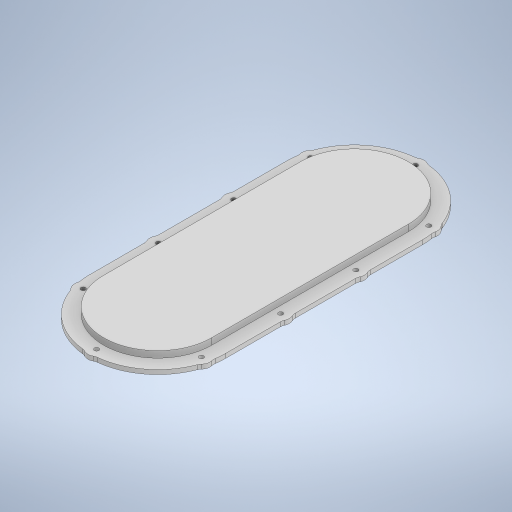
# Autodesk Inventor part: top_housing_bottom_plate
Saved by Autodesk Inventor 2023.1 (Build 271208000, 208)
## iProperties
Created: 2026-04-22
Part Number: top_housing_bottom_plate
Material: Generic
Document SubType Name: Modeling
Designer: Lars
Density: 1 g/cm^3
Appearance: Default
Author: Lars
Autodesk Inventor part; units mm, degrees
ref_plane "YZ Plane" through (0, 0, 0) normal (1, 0, 0) x (0, 1, 0)
ref_plane "XZ Plane" through (0, 0, 0) normal (0, 1, 0) x (-1, 0, 0)
ref_plane "XY Plane" through (0, 0, 0) normal (0, 0, 1) x (1, 0, 0)
sketch "Sketch2" plane through (0, 0, 0) normal (0, 1, 0) x (-1, 0, 0)
  line L0 (15, -6.5) -> (-46, -6.5) construction
  line L1 (-46, -6.5) -> (-46, -90.5) construction
  line L2 (-46, -90.5) -> (15, -90.5) construction
  line L3 (15, -90.5) -> (15, -6.5) construction
  line L4 (46, 27.1) -> (14, 27.1) construction
  line L5 (14, 27.1) -> (14, 11.1) construction
  line L6 (14, 11.1) -> (46, 11.1) construction
  line L7 (46, 11.1) -> (46, 27.1) construction
  line L8 (9, 32.5) -> (-40, 32.5) construction
  line L9 (-40, 32.5) -> (-40, 90.5) construction
  line L10 (-40, 90.5) -> (9, 90.5) construction
  line L11 (9, 90.5) -> (9, 32.5) construction
  line L12 (-15.5, -6.5) -> (-15.5, -90.5) construction
  line L13 (-15.5, 32.5) -> (-15.5, 90.5) construction
  line L14 (-46, -90.5) -> (46, -90.5) construction
  line L15 (46, -90.5) -> (46, 90.5) construction
  line L16 (46, 90.5) -> (-46, 90.5) construction
  line L17 (-46, 90.5) -> (-46, -90.5) construction
  line L18 (46, 0) -> (-46, 0) construction
  line L19 (-62.5, 267) -> (62.5, 267) construction
  line L20 (62.5, 267) -> (62.5, -267) construction
  line L21 (62.5, -267) -> (-62.5, -267) construction
  line L22 (-62.5, -267) -> (-62.5, 267) construction
  line L23 (62.5, 0) -> (-62.5, 0) construction
  circle A0 centre (46, 11.1) radius 1.5
  circle A1 centre (14, 27.1) radius 1.5
  circle A2 centre (9, 32.5) radius 1.5
  circle A3 centre (-40, 32.5) radius 1.5
  circle A4 centre (9, 90.5) radius 1.5
  circle A5 centre (-40, 90.5) radius 1.5
  circle A6 centre (15, -6.5) radius 1.5
  circle A7 centre (15, -90.5) radius 1.5
  circle A8 centre (-46, -90.5) radius 1.5
  circle A9 centre (-46, -6.5) radius 1.5
  line L24 (0, 142) -> (0, 142)
  line L25 (-50, 92) -> (-50, 0)
  line L26 (-50, 0) -> (50, 0) construction
  line L27 (50, 0) -> (50, 92)
  line L28 (50, 0) -> (-50, 0) construction
  line L29 (-50, 0) -> (-50, -90)
  line L30 (0, -140) -> (0, -140)
  line L31 (50, -90) -> (50, 0)
  arc A10 (50, 92) -> (0, 142) centre (0, 92) ccw
  arc A11 (0, 142) -> (-50, 92) centre (0, 92) ccw
  arc A12 (-50, -90) -> (0, -140) centre (0, -90) ccw
  arc A13 (0, -140) -> (50, -90) centre (0, -90) ccw
  line L32 (63, 92) -> (63, 0)
  line L33 (63, 0) -> (63, -90)
  arc A14 (0, -153) -> (63, -90) centre (0, -90) ccw
  arc A15 (-63, -90) -> (0, -153) centre (0, -90) ccw
  line L34 (-63, -90) -> (-63, 0)
  line L35 (-63, 0) -> (-63, 92)
  arc A16 (0, 155) -> (-63, 92) centre (0, 92) ccw
  arc A17 (63, 92) -> (0, 155) centre (0, 92) ccw
  line L36 (56.5, 92) -> (56.5, 0) construction
  line L37 (56.5, 0) -> (56.5, -90) construction
  arc A18 (0, -146.5) -> (56.5, -90) centre (0, -90) ccw construction
  arc A19 (-56.5, -90) -> (0, -146.5) centre (0, -90) ccw construction
  line L38 (-56.5, -90) -> (-56.5, 0) construction
  line L39 (-56.5, 0) -> (-56.5, 92) construction
  arc A20 (0, 148.5) -> (-56.5, 92) centre (0, 92) ccw construction
  arc A21 (56.5, 92) -> (0, 148.5) centre (0, 92) ccw construction
  circle A22 centre (0, -146.5) radius 2.05
  circle A23 centre (0, -146.5) radius 8.05
  circle A24 centre (54.6727, -104.253) radius 2.05
  circle A25 centre (54.6727, -104.253) radius 8.05
  circle A26 centre (56.5, -34.95) radius 2.05
  circle A27 centre (56.5, -34.95) radius 8.05
  circle A28 centre (56.5, 34.7508) radius 2.05
  circle A29 centre (56.5, 34.7508) radius 8.05
  circle A30 centre (0, 148.5) radius 2.05
  circle A31 centre (0, 148.5) radius 8.05
  circle A32 centre (54.6727, 106.253) radius 2.05
  circle A33 centre (54.6727, 106.253) radius 8.05
  line L40 (0, -153) -> (0, -140) construction
  circle A34 centre (-54.6727, -104.253) radius 2.05
  circle A35 centre (-54.6727, -104.253) radius 8.05
  circle A36 centre (-56.5, -34.95) radius 2.05
  circle A37 centre (-56.5, -34.95) radius 8.05
  circle A38 centre (-56.5, 34.7508) radius 2.05
  circle A39 centre (-56.5, 34.7508) radius 8.05
  circle A40 centre (-54.6727, 106.253) radius 2.05
  circle A41 centre (-54.6727, 106.253) radius 8.05
  circle A42 centre (0, -90) radius 5
  circle A43 centre (0, 92) radius 5
  circle A44 centre (0, 0) radius 5
  point P0 (-50, 142)
  point P1 (-50, -140)
  point P2 (0, -140)
  point P3 (0, 142)
  point P4 (5.0107, -152.8004)
  point P5 (59.5053, -110.691)
  point P6 (62.0334, -100.9937)
  point P7 (63, -39.6989)
  point P8 (63, -30.2011)
  point P9 (63, 30.0019)
  point P10 (63, 39.4997)
  point P11 (62.0334, 102.9937)
  point P12 (59.5053, 112.691)
  point P13 (5.0107, 154.8004)
  point P14 (-5.0107, 154.8004)
  point P15 (-59.5053, 112.691)
  point P16 (-62.0334, 102.9937)
  point P17 (-63, 39.4997)
  point P18 (-63, 30.0019)
  point P19 (-63, -30.2011)
  point P20 (-63, -39.6989)
  point P21 (-62.0334, -100.9937)
  point P22 (-59.5053, -110.691)
  point P23 (-5.0107, -152.8004)
  dimension "d9" = 61
  dimension "d10" = 84
  dimension "d11" = 32
  dimension "d12" = 16
  dimension "d13" = 49
  dimension "d14" = 58
  dimension "d15" = 39
  dimension "d16" = 5.4
  dimension "d17" = 5
  dimension "d18" = 125
  dimension "d19" = 534
  dimension "d20" = 3
  dimension "d21" = 3
  dimension "d22" = 3
  dimension "d23" = 3
  dimension "d24" = 3
  dimension "d25" = 3
  dimension "d26" = 3
  dimension "d27" = 3
  dimension "d28" = 3
  dimension "d29" = 3
  dimension "d33" = 100
  dimension "d34" = 142
  dimension "d36" = 140
  dimension "d37" = 50
  dimension "d38" = 13
  dimension "d43" = 6.5
  dimension "d44" = 4.1
  dimension "d45" = 6
  dimension "d48" = 75.388
  dimension "d50" = 4.1
  dimension "d51" = 6
  dimension "d52" = 34.95
  dimension "d53" = 4.1
  dimension "d54" = 6
  dimension "d55" = 34.7508
  dimension "d56" = 4.1
  dimension "d57" = 6
  dimension "d60" = 75.388
  dimension "d63" = 10
  dimension "d64" = 10
  dimension "d65" = 10
  constraints: 82 end point, 45 centre point, 24 point on circle, 19 coincident, 18 parallel, 11 midpoint, 9 point on line, 8 tangent, 7 horizontal, 7 perpendicular, 5 symmetric about line, 3 equal radius, 33 other
  measures "d9" distance of L2.end L1.end
  measures "d10" distance of L1.end L0.end
  measures "d11" distance of L6.end L5.end
  measures "d12" distance of L5.end L4.end
  measures "d13" distance of L9.end L10.end
  measures "d14" distance of L8.end L9.end
  measures "d15" distance between parallel lines of L0 L8
  measures "d16" distance between parallel lines of L4 L8
  measures "d17" distance between parallel lines of L11 L5
  measures "d18" distance of L20.end L21.end
  measures "d19" distance of L19.end L20.end
  measures "d20" diameter of A0
  measures "d21" diameter of A1
  measures "d22" diameter of A2
  measures "d23" diameter of A3
  measures "d24" diameter of A4
  measures "d25" diameter of A5
  measures "d26" diameter of A6
  measures "d27" diameter of A7
  measures "d28" diameter of A8
  measures "d29" diameter of A9
  measures "d33" distance of L26.end L25.end
  measures "d34" distance of L25.end point (-50, 142)
  measures "d36" distance of L25.end point (-50, -140)
  measures "d37" radius of A10
  measures "d38" distance between parallel lines of L27 L32
  measures "d43" distance between parallel lines of L27 L36
  measures "d44" diameter of A22
  measures "d45" radial gap between concentric circles of A22 A23
  measures "d50" diameter of A26
  measures "d51" radial gap between concentric circles of A26 A27
  measures "d52" distance from line of L23 A26.centre
  measures "d53" diameter of A28
  measures "d54" radial gap between concentric circles of A28 A29
  measures "d55" distance from line of L23 A28.centre
  measures "d56" diameter of A30
  measures "d57" radial gap between concentric circles of A30 A31
  measures "d63" diameter of A42
  measures "d64" diameter of A43
  measures "d65" diameter of A44
extrude "Extrusion1" add sketch "Sketch2" along normal blind 6 contours A0 | A1 | A2 | A3 | A4 | A5 | A6 | A7 | A8 | A9 | A11 A41 A31 A10 A33 L27 A29 L31 A27 A13 A25 A23 A12 A35 L29 A37 L25 A39 | A39 L25 | A11 A41 | A11 A10 A31 | A37 L29 | A10 A33 | A35 A12 | L27 A29 | A23 A13 A12 | A25 A13 | L31 A27 | A42 | A43 | A44
extrude "Extrusion2" add sketch "Sketch2" against normal blind 4 contours A0 | A1 | A2 | A3 | A4 | A5 | A6 | A7 | A8 | A9 | A11 A41 A31 A10 A33 L27 A29 L31 A27 A13 A25 A23 A12 A35 L29 A37 L25 A39 | L25 A39 L35 A16 A41 A11 | A39 L25 | L25 A39 L35 | A41 A16 A11 | A11 A41 | L25 L29 A37 L34 L35 A39 | L35 A39 | A41 A16 A31 A11 | A41 A16 | A31 A16 A17 A10 A11 | A11 A10 A31 | A37 L29 | L29 A37 L34 | A31 A17 A16 | A31 A17 A33 A10 | L29 A12 A35 A15 L34 A37 | L34 A37 | A33 A17 A10 | A10 A33 | A33 A17 | A33 A17 L32 A29 L27 A10 | A35 A12 | A12 A35 A15 | A12 A23 A15 A35 | A15 A35 | A29 L32 L27 | L27 A29 | A23 A13 A12 | A12 A13 A23 A14 A15 | A29 L32 | A29 L32 L33 A27 L31 L27 | A13 A25 A14 A23 | A15 A14 A23 | A25 A13 | A13 A25 A14 | A27 L33 L31 | L31 A27 | A13 L31 A27 L33 A14 A25 | A14 A25 | A27 L33 | A42 | A43 | A44
fillet "Fillet1" radius 8 20 edges at (-5.0107, -2, -152.8004) (-59.5053, -2, -110.691) (-62.0334, -2, -100.9937) (-63, -2, -39.6989) (-63, -2, -30.2011) (-63, -2, 30.0019) (-63, -2, 39.4997) (-62.0334, -2, 102.9937) (-59.5053, -2, 112.691) (-5.0107, -2, 154.8004) (5.0107, -2, 154.8004) (59.5053, -2, 112.691) (62.0334, -2, 102.9937) (63, -2, 39.4997) (62.0334, -2, -100.9937) (63, -2, -30.2011) (59.5053, -2, -110.691) (63, -2, -39.6989) (63, -2, 30.0019) (5.0107, -2, -152.8004)
sketch "Sketch3" plane through (0, 0, 0) normal (0, 1, 0) x (1, 0, 0)
  point P0 (0, 0)
equation "\"d43\" = 0.5 * d38"
body "Solid1"
